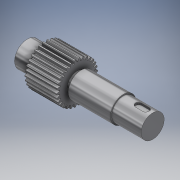
# Autodesk Inventor part: Keyway Slot on Shaft
Saved by Autodesk Inventor 2018.2 (Build 222227000, 227)
## iProperties
Created: 2013-11-18
Part Number: Keyway Slot on Shaft
Material: Generic
Document SubType Name: Modeling
Designer: normanpa
Density: 1 g/cm^3
Appearance: Cadet Blue
Author: normanpa
Autodesk Inventor part; units mm, degrees
ref_plane "YZ Plane" through (0, 0, 0) normal (1, 0, 0) x (0, 1, 0)
sketch "Sketch1" plane through (0, 0, 0) normal (0, 0, 1) x (1, 0, 0)
  line L0 (0, 0) -> (24, 0)
  line L1 (0, 35) -> (0, 50)
  line L2 (0, 50) -> (24, 50)
  line L3 (24, 50) -> (24, 20)
  line L4 (24, 20) -> (18, 20)
  line L5 (18, 20) -> (18, 35)
  line L6 (18, 35) -> (0, 35)
  dimension "d0" = 100
  dimension "d1" = 70
  dimension "d2" = 24
  dimension "d3" = 18
  dimension "d4" = 40
  constraints: 14 end point, 5 perpendicular, 1 horizontal, 1 parallel, 1 vertical, 1 vertical alignment
  measures "d0" diameter of L2 L0
  measures "d1" diameter of L6 L0
  measures "d2" distance of L1.end L2.end
  measures "d3" distance between parallel lines of L5 L1
  measures "d4" diameter of L4 L0
revolve "Revolution1" add sketch "Sketch1" angle 360 about axis through (0, 0, 0) along (1, 0, 0)
thread "Thread1" size "M70x6" class "6H" standard "ANSI Metric M Profile" full length
ref_plane "Work Plane1" through (12, 50, 0) normal (0, 1, 0) x (-1, 0, 0)
sketch "Sketch2" plane through (12, 50, 0) normal (0, 1, 0) x (-1, 0, 0)
  line L0 (12, 50) -> (12, -50) projected
  line L1 (-12, 50) -> (-12, -50) projected
  line L2 (-12, 20) -> (-12, -20) projected
  line L3 (-12, 0) -> (12, 0)
  point P0 (0, 0)
  constraints: 2 end point, 2 midpoint, 1 perpendicular
hole "Hole1" at (12, 50, 0) direction (0, -1, 0) diameter 10 depth 8
pattern_circular "Circular Pattern1" count 3 over 360 about axis through (12, 0, 0) along (1, 0, 0) of "Hole1"
chamfer "Chamfer1" distance 2 angle 45 2 edges at (0, -50, 0) (24, -50, 0)
sketch "Sketch3" plane through (0, 0, 0) normal (0, 0, 1) x (1, 0, 0)
  line L0 (-91, -16) -> (-97, -16)
  line L1 (-97, -20) -> (-97, -16)
  line L2 (-41, -32) -> (-91, -32)
  line L3 (-91, -32) -> (-91, -16)
  line L4 (-97, -20) -> (-119, -20)
  line L5 (-119, 0) -> (-119, -20)
  line L6 (-119, 0) -> (-119, -20)
  line L7 (-41, -32) -> (-41, -16)
  line L8 (-41, -16) -> (-35, -16)
  line L9 (-35, -16) -> (-35, -20)
  line L10 (77, 0) -> (-119, 0)
  line L11 (31, -20) -> (31, -18)
  line L12 (-35, -20) -> (31, -20)
  line L13 (31, -18) -> (77, -18)
  line L14 (77, -18) -> (77, 0)
  line L15 (24, 48) -> (24, -48) projected
  point P0 (0, 0)
  dimension "d21" = 40
  dimension "d22" = 22
  dimension "d23" = 6
  dimension "d24" = 50
  dimension "d25" = 6
  dimension "d26" = 66
  dimension "d27" = 46
  dimension "d28" = 32
  dimension "d29" = 64
  dimension "d30" = 40
  dimension "d31" = 36
  dimension "d33" = 53
  constraints: 31 end point, 13 perpendicular, 2 coincident, 2 collinear, 1 parallel, 1 point on line, 1 vertical
  measures "d21" diameter of L4 L10
  measures "d22" distance between parallel lines of L1 L5
  measures "d23" distance of L3.end L0.end
  measures "d24" distance between parallel lines of L7 L3
  measures "d25" distance of L7.end L8.end
  measures "d26" distance between parallel lines of L11 L9
  measures "d27" distance between parallel lines of L14 L11
  measures "d28" diameter of L0 L10
  measures "d29" diameter of L2 L10
  measures "d30" diameter of L12 L10
  measures "d31" diameter of L13 L10
  measures "d33" distance between parallel lines of L15 L14
revolve "Revolution2" add sketch "Sketch3" angle 360 about axis through (77, 0, 0) along (-1, 0, 0) separate body
sketch "Sketch4" plane through (-41, 0, 0) normal (1, 0, 0) x (0, 0, -1)
  circle A0 centre (0, 0) radius 32 projected
  circle A1 centre (0, 0) radius 27.5
  arc A2 (-0.75, 27.4898) -> (-2.5, 31.9022) centre (-12.3222, 25.4534) ccw
  arc A3 (2.5, 31.9022) -> (0.75, 27.4898) centre (12.3222, 25.4534) ccw
  dimension "d35" = 55
  dimension "d37" = 2.5
  dimension "d38" = 2.5
  dimension "d39" = 0.75
  dimension "d40" = 0.75
  dimension "d41" = 11.75
  constraints: 8 point on circle, 3 centre point, 1 coincident, 1 equal radius
  measures "d35" diameter of A1
  measures "d37" horizontal distance of A0.centre A0.start
  measures "d38" horizontal distance of A0.centre A0.end
  measures "d39" horizontal distance of A0.centre A1.start
  measures "d40" horizontal distance of A0.centre A1.end
  measures "d41" radius of A2
extrude "Extrusion1" cut sketch "Sketch4" against normal up to next contours A3 A1 A2 A0 picked at (-0.3772, 30.022)
pattern_circular "Circular Pattern2" count 30 over 360 about axis through (-66, 0, 0) along (-1, 0, 0) of "Extrusion1"
ref_plane "Work Plane2" through (54, 18, 0) normal (0, 1, 0) x (-1, 0, 0)
sketch "Sketch5" plane through (54, 18, 0) normal (0, 1, 0) x (-1, 0, 0)
  line L0 (-23, -18) -> (-23, 18) projected
  line L1 (-1, 0) -> (-13, 0) construction
  line L2 (-1, 5) -> (-13, 5)
  line L3 (-13, -5) -> (-1, -5)
  arc A0 (-1, -5) -> (-1, 5) centre (-1, 0) ccw
  arc A1 (-13, 5) -> (-13, -5) centre (-13, 0) ccw
  point P0 (54, 0)
  point P1 (-7, 0)
  point P2 (-23, 0)
  dimension "d47" = 12
  dimension "d48" = 10
  dimension "d49" = 10
  constraints: 8 end point, 4 point on circle, 4 tangent, 2 centre point, 2 midpoint, 1 horizontal, 1 horizontal alignment, 1 parallel
  measures "d47" distance of L1.start L1.end
  measures "d48" diameter of A1
  measures "d49" distance of point (-23, 0) L1.end
extrude "Extrusion2" cut sketch "Sketch5" against normal blind 3.5
equation "\"d38\" = d37"
equation "\"d40\" = d39"
body "Solid1"
body "Solid2"
